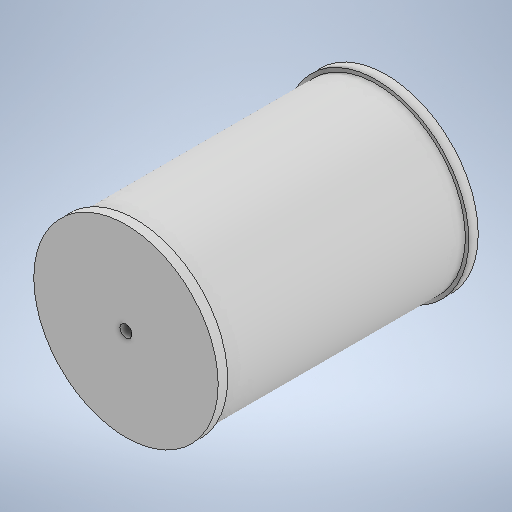
# Autodesk Inventor part: 13042026-14
Saved by Autodesk Inventor 2025.2 (Build 292293000, 293)
## iProperties
Created: 2026-04-14
Part Number: 13042026-14
Material: Generic
Document SubType Name: Modeling
Designer: Oski
Density: 1 g/cm^3
Appearance: Default
Author: Oski
Autodesk Inventor part; units mm, degrees
ref_plane "YZ Plane" through (0, 0, 0) normal (1, 0, 0) x (0, 1, 0)
ref_plane "XZ Plane" through (0, 0, 0) normal (0, 1, 0) x (-1, 0, 0)
ref_plane "XY Plane" through (0, 0, 0) normal (0, 0, 1) x (1, 0, 0)
sketch "Sketch1" plane through (0, 0, 0) normal (0, 0, 1) x (1, 0, 0)
  circle A0 centre (0, 0) radius 37.5
  dimension "d0" = 75
  constraints: 2 coincident, 1 centre point
  measures "d0" diameter of A0
extrude "Extrusion1" add sketch "Sketch1" along normal mid plane 110
sketch "Sketch5" plane through (0, 0, 55) normal (0, 0, 1) x (1, 0, 0)
  circle A0 centre (0, 0) radius 39
  dimension "d22" = 78
  constraints: 1 centre point, 1 coincident
  measures "d22" diameter of A0
extrude "Extrusion4" add sketch "Sketch5" against normal blind 4
mirror "Mirror2" about plane through (0, 0, 0) normal (0, 0, 1) of "Extrusion4"
sketch "Sketch4" plane through (0, 0, -55) normal (0, 0, -1) x (-1, 0, 0)
  point P0 (0, 0)
  point P1 (0, 0)
  constraints: 1 coincident
hole "Hole1" at (0, 0, -55) direction (0, 0, 1) diameter 26 depth 40 counterbore diameter 30.2 counterbore depth 9.3
sketch "Sketch6" plane through (0, 0, 55) normal (0, 0, 1) x (1, 0, 0)
  circle A0 centre (0, 0) radius 2.55
  dimension "d25" = 5.1
  constraints: 1 centre point, 1 coincident
  measures "d25" diameter of A0
extrude "Extrusion5" cut sketch "Sketch6" against normal blind 10
sketch "Sketch7" plane through (0, 0, 55) normal (0, 0, 1) x (1, 0, 0)
  circle A0 centre (0, 0) radius 2.55 projected
  line L0 (-1.5, -2.0622) -> (-1.5, 2.0622)
  line L1 (1.5, 2.0622) -> (1.5, -2.0622)
  arc A1 (-1.5, -2.0622) -> (1.5, -2.0622) centre (0, 0) ccw
  arc A2 (1.5, 2.0622) -> (-1.5, 2.0622) centre (0, 0) ccw
  dimension "d28" = 1.5
  constraints: 9 point on circle, 4 end point, 2 centre point, 2 coincident, 2 parallel, 1 vertical
  measures "d28" distance from line of L0 point (0, 0)
extrude "Extrusion6" cut sketch "Sketch7" against normal through all contours L1 A0 L0
body "Solid1"
